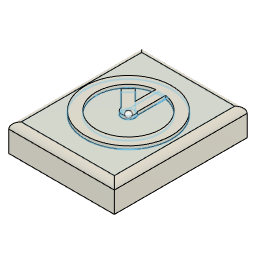
CO2buttn v6 (Autodesk Fusion 360 design; units mm, degrees)
Autodesk Fusion 360 part; units mm, degrees
sketch "Sketch1" plane through (0, 0, 0) normal (0, 1, 0) x (1, 0, 0)
  line L0 (0, 0) -> (13.5, 0)
  line L1 (13.5, 0) -> (13.5, 17)
  line L2 (13.5, 17) -> (0, 17)
  line L3 (0, 17) -> (0, 0)
  dimension "d1" = 17
  dimension "d2" = 13.5
  constraint horizontal L0
  constraint vertical L1
  constraint horizontal L2
  constraint vertical L3
  constraint coincident L0.start L3.end
  measures "d1" distance of L0.start L2.end
  measures "d2" distance of L1.end L2.end
extrude "Extrude1" add sketch "Sketch1" along normal blind 3.5
shell "Shell1" thickness 0.8 removed faces 1 at (4.5, 0, -11.3333)
fillet "Fillet1" radius 0.8 4 edges at (6.75, 3.5, 0) (0, 3.5, -8.5) (6.75, 3.5, -17) (13.5, 3.5, -8.5)
sketch "Sketch2" plane through (0, 3.5, 0) normal (0, 1, 0) x (-1, 0, 0)
  line L0 (-12.7, -16.2) -> (-0.8, -16.2)
  line L1 (-0.8, -16.2) -> (-0.8, -0.8)
  line L2 (-0.8, -0.8) -> (-12.7, -0.8)
  line L3 (-12.7, -0.8) -> (-12.7, -16.2)
  circle A0 centre (-6.8051, -8.5) radius 5.5188
  circle A1 centre (-6.8051, -8.5) radius 4.1313
  line L4 (-6.2112, -12.8845) -> (-7.4916, -12.8845)
  line L5 (-7.4916, -12.8845) -> (-7.4916, -8.2604)
  line L6 (-7.4916, -8.2604) -> (-6.2112, -8.2604)
  line L7 (-6.2112, -8.2604) -> (-6.2112, -12.8845)
  line L8 (-4.7993, -11.3803) -> (-7.4152, -8.7643)
  line L9 (-7.4152, -8.7643) -> (-6.5099, -7.8589)
  line L10 (-6.5099, -7.8589) -> (-3.8939, -10.4749)
  line L11 (-3.8939, -10.4749) -> (-4.7993, -11.3803)
  circle A2 centre (-6.8051, -8.5) radius 0.8328
  constraint concentric A0 A1
  constraint horizontal L4
  constraint vertical L5
  constraint horizontal L6
  constraint vertical L7
  constraint concentric A1 A2
extrude "Extrude4" add sketch "Sketch2" along normal blind 0.4 contours A0 | A1 L5 L7 L8 A2 | A1 L4 L5 L7 | L5 L6 L9 L10 A2 | L5 L6 L8 L9 A2 | L7 L8 A2 | L7 L8 L10 L11 A2 | L6 L7 L9 L10 A2 | L6 L7 L8 L9 A2
